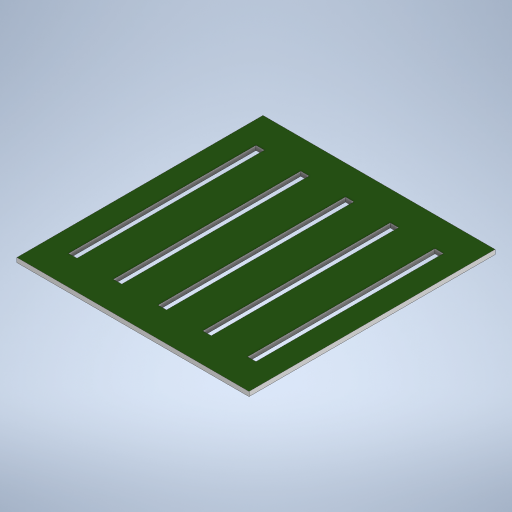
# Autodesk Inventor part: TopPCB
Saved by Autodesk Inventor 2023 (Build 270158000, 158)
## iProperties
Created: 2024-03-19
Part Number: TopPCB
Material: Generic
Document SubType Name: Modeling
Designer: noname
Density: 1 g/cm^3
Appearance: Default
Author: noname
Autodesk Inventor part; units mm, degrees
ref_plane "YZ Plane" through (0, 0, 0) normal (1, 0, 0) x (0, 1, 0)
ref_plane "XZ Plane" through (0, 0, 0) normal (0, 1, 0) x (-1, 0, 0)
ref_plane "XY Plane" through (0, 0, 0) normal (0, 0, 1) x (1, 0, 0)
sketch "Sketch1" plane through (0, 0, 0) normal (0, 1, 0) x (-1, 0, 0)
  line L0 (0, 0) -> (-83, 0)
  line L1 (-83, 0) -> (-83, -88)
  line L2 (-83, -88) -> (0, -88)
  line L3 (0, -88) -> (0, 0)
  line L4 (-8, -77.5) -> (-11, -77.5)
  line L5 (-11, -77.5) -> (-11, -10.5)
  line L6 (-11, -10.5) -> (-8, -10.5)
  line L7 (-8, -10.5) -> (-8, -77.5)
  line L8 (-24, -77.5) -> (-27, -77.5)
  line L9 (-27, -77.5) -> (-27, -10.5)
  line L10 (-27, -10.5) -> (-24, -10.5)
  line L11 (-24, -10.5) -> (-24, -77.5)
  line L12 (-40, -77.5) -> (-43, -77.5)
  line L13 (-43, -77.5) -> (-43, -10.5)
  line L14 (-43, -10.5) -> (-40, -10.5)
  line L15 (-40, -10.5) -> (-40, -77.5)
  line L16 (-56, -77.5) -> (-59, -77.5)
  line L17 (-59, -77.5) -> (-59, -10.5)
  line L18 (-59, -10.5) -> (-56, -10.5)
  line L19 (-56, -10.5) -> (-56, -77.5)
  line L20 (-72, -77.5) -> (-75, -77.5)
  line L21 (-75, -77.5) -> (-75, -10.5)
  line L22 (-75, -10.5) -> (-72, -10.5)
  line L23 (-72, -10.5) -> (-72, -77.5)
  point P0 (-8, -44)
  point P1 (0, -44)
  point P2 (-24, -44)
  point P3 (-40, -44)
  point P4 (-56, -44)
  point P5 (-72, -44)
  dimension "d1" = 88
  dimension "d2" = 3
  dimension "d3" = 67
  dimension "d4" = 8
  dimension "d7" = 16
  dimension "d12" = 8
  constraints: 48 end point, 4 parallel, 3 horizontal, 2 midpoint, 2 perpendicular, 1 horizontal alignment, 36 other
  measures "d1" distance between parallel lines of L0 L2
  measures "d2" distance between parallel lines of L5 L7
  measures "d3" distance between parallel lines of L4 L6
  measures "d4" distance between parallel lines of L3 L7
  measures "d7" distance of L4.start L8.start
  measures "d12" distance between parallel lines of L1 L21
extrude "Extrusion1" add sketch "Sketch1" along normal blind 1.6
body "Solid1"
